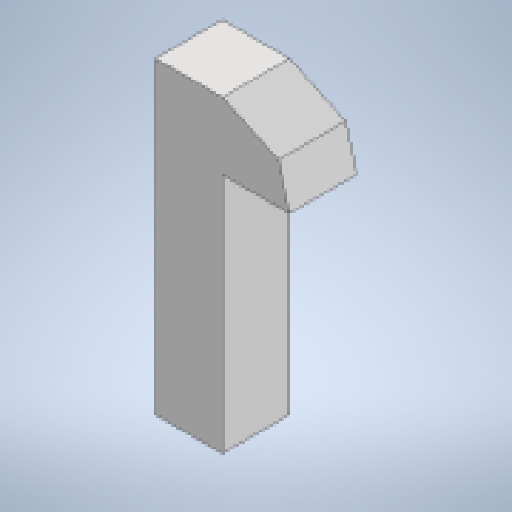
# Autodesk Inventor part: calle
Saved by Autodesk Inventor 2024 (Build 280153000, 153)
## iProperties
Created: 2024-03-24
Part Number: calle
Material: Générique
Document SubType Name: Modeling
Designer: phaly
Density: 1 g/cm^3
Appearance: Par défaut
Author: phaly
Autodesk Inventor part; units mm, degrees
ref_plane "YZ Plane" through (0, 0, 0) normal (1, 0, 0) x (0, 1, 0)
ref_plane "XZ Plane" through (0, 0, 0) normal (0, 1, 0) x (-1, 0, 0)
ref_plane "XY Plane" through (0, 0, 0) normal (0, 0, 1) x (1, 0, 0)
sketch "Esquisse1" plane through (0, 0, 0) normal (0, 0, 1) x (1, 0, 0)
  line L0 (0, 0) -> (0, 23)
  line L1 (-2, 0) -> (12, 0) projected
  line L2 (0, -4.6) -> (0, 27.6) projected
  line L3 (0, 23) -> (5, 23)
  line L4 (5, 23) -> (9.1829, 21.0495)
  line L5 (9.1829, 21.0495) -> (10, 18)
  line L6 (10, 18) -> (5, 18)
  line L7 (5, 18) -> (5, 0)
  line L8 (0, 0) -> (5, 0)
  point P0 (0, 0)
  dimension "d8" = 5
  dimension "d9" = 5
  dimension "d10" = 75
  dimension "d12" = 130
  dimension "d13" = 18
  dimension "d14" = 5
  dimension "d24" = 5
  constraints: 14 end point, 2 collinear, 2 perpendicular, 1 midpoint, 1 parallel, 1 point on line
  measures "d8" distance of L5.end L6.end
  measures "d9" distance of point (0, 0) L7.end
  measures "d10" angle of L6 L5
  measures "d12" angle of L5 L4
  measures "d13" distance of L6.end L7.end
  measures "d14" distance of L0.end L3.end
  measures "d24" distance of L6.end L3.end
extrude "Extrusion1" add sketch "Esquisse1" along normal blind 5
sketch "Esquisse3" plane through (0, 0, 0) normal (0, -1, 0) x (1, 0, 0)
  line L0 (0, 5) -> (5, 5) projected
  line L1 (0, 0) -> (0, 5) projected
  point P0 (2.5, 2.5)
  point P1 (2.5, 5)
  dimension "d15" = 2.5
  dimension "d16" = 2.5
  constraints: 1 midpoint
  measures "d15" distance of point (2.5, 5) point (2.5, 2.5)
  measures "d16" distance from line of L1 point (2.5, 2.5)
hole "Perçage1" at (2.5, 0, 2.5) direction (0, 1, 0) diameter 2 depth 8 tip angle 118
